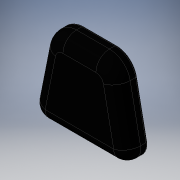
# Autodesk Inventor part: SCHUNK-1352153-Fingereinsatz Typ A Co-act EGP-C
Saved by Autodesk Inventor 2019 (Build 230136000, 136)
## iProperties
Created: 2022-08-31
Part Number: SCHUNK-1352153-Fingereinsatz Typ A Co-act EGP-C
Material: Generic
Catalog Web Link: www.cadenas.de
Description: EIS Co-act EGP-Fingereinsatz Co-act EGP
Vendor: SCHUNK
Document SubType Name: Modeling
Designer: psAdmin
Manufacturer: SCHUNK
Mass: 1.77604 g
Surface Area: 10.2019 cm^2
Volume: 1.77604 cm^3
Density: 1 g/cm^3
Appearance: PSOLRGB-50-50-50
Category: PARTsolutions
Company: SCHUNK
Title: SCHUNK-1352153-Fingereinsatz Typ A Co-act EGP-C
Author: Cadenas PARTsolutions
Comments: Fingereinsatz Co-act EGP
PSOL_IDENT_0: {$CADENAS_DATA/23d-libs/schunk/greifsysteme/greifmodule/co_act/co_act_egp_c/eis_co_act_egp.prj},242
PSOL_IDENT_1: {VTYP=3D},{NB=SCHUNK-1352153-Fingereinsatz Typ A Co-act EGP-C},{LINA=SCHUNK-1352153-Fingereinsatz Ty
PSOL_IDENT_2: p A Co-act EGP-C},{NN=EIS Co-act EGP},{DATE=21.12.2021 12:23:17},{GEOMDATE=21.11.2018 07:09:32},{VER
PSOL_IDENT_3: SION=},{LINEID=80},{WBVAR=},{WBNUMERIC=}  {NB=SCHUNK-1352153-Fingereinsatz Typ A Co-act EGP-C},{LINA=
PSOL_IDENT_4: SCHUNK-1352153-Fingereinsatz Typ A Co-act EGP-C},{KT=DUMMY},{IDNR=1352153},{TYP=Fingereinsatz Typ A
PSOL_IDENT_5: Co-act EGP-C},{TYP1=1.000},{L=5.000},{B=24.000},{H=20.000},{B1=8.000},{R1=5.000},{R2=3.200},{R3=0.50
PSOL_IDENT_6: 0},{R4=0.000},{AA=0.000},{TA=0.000},{RA=0.000},{AA2=0.000},{TA2=0.000},{RA2=0.000},{AKR=0.000},{TKR=
PSOL_IDENT_7: 0.000},{BR=0.000},{AR=0.000},{ABRI=0.000}
NB: SCHUNK-1352153-Fingereinsatz Typ A Co-act EGP-C
NN: EIS Co-act EGP
NT: Fingereinsatz Co-act EGP
NBSYN: SCHUNK-$IDNR.-$TYP.
LINA: SCHUNK-1352153-Fingereinsatz Typ A Co-act EGP-C
CATALOG: SCHUNK
IDNR: 1352153
TYP: Fingereinsatz Typ A Co-act EGP-C
TYP1: 1
L: 5
B: 24
H: 20
B1: 8
R1: 5
R2: 3.2
R3: 0.5
R4: 0
AA: 0
TA: 0
RA: 0
AA2: 0
TA2: 0
RA2: 0
AKR: 0
TKR: 0
BR: 0
AR: 0
ABRI: 0
SUPPLIER: SCHUNK
ARTICLENO: SCHUNK-1352153-Fingereinsatz Typ A Co-act EGP-C
BOMINFO: SCHUNK-1352153-Fingereinsatz Typ A Co-act EGP-C
CREATOR: CADENAS GmbH
Autodesk Inventor part; units mm, degrees
sketch "Sketch_1" plane through (0, 0, 0) normal (0, 0, 1) x (1, 0, 0)
  arc A0 (-11.2345, -6.1724) -> (-8.0966, -10) centre (-8.0966, -6.8) ccw
  line L0 (-8.0966, -10) -> (8.0966, -10)
  arc A1 (8.0966, -10) -> (11.2345, -6.1724) centre (8.0966, -6.8) ccw
  line L1 (11.2345, -6.1724) -> (8.8039, 5.9806)
  arc A2 (8.8039, 5.9806) -> (3.901, 10) centre (3.901, 5) ccw
  line L2 (3.901, 10) -> (-3.901, 10)
  arc A3 (-3.901, 10) -> (-8.8039, 5.9806) centre (-3.901, 5) ccw
  line L3 (-8.8039, 5.9806) -> (-11.2345, -6.1724)
  constraints: 8 end point, 8 point on circle, 4 centre point
extrude "Extrusion1" add sketch "Sketch_1" along normal blind 5
fillet "Fillet1" radius 3.2 8 edges at (-10.5713, -8.8288, 5) (0, -10, 5) (10.5713, -8.8288, 5) (10.0192, -0.0959, 5) (7.0709, 8.8667, 5) (0, 10, 5) (-7.0709, 8.8667, 5) (-10.0192, -0.0959, 5)
fillet "Fillet2" radius 0.5 8 edges at (-10.5713, -8.8288, 0) (-10.0192, -0.0959, 0) (-7.0709, 8.8667, 0) (0, 10, 0) (7.0709, 8.8667, 0) (10.0192, -0.0959, 0) (10.5713, -8.8288, 0) (0, -10, 0)
ref_plane "EIS_XY" through (0, 0, 0) normal (0, 0, 1) x (1, 0, 0)
ref_plane "EIS_YZ" through (0, 0, 0) normal (1, 0, 0) x (0, 1, 0)
ref_plane "EIS_ZX" through (0, 0, 0) normal (0, 1, 0) x (0, 0, 1)
body "Solid1"
